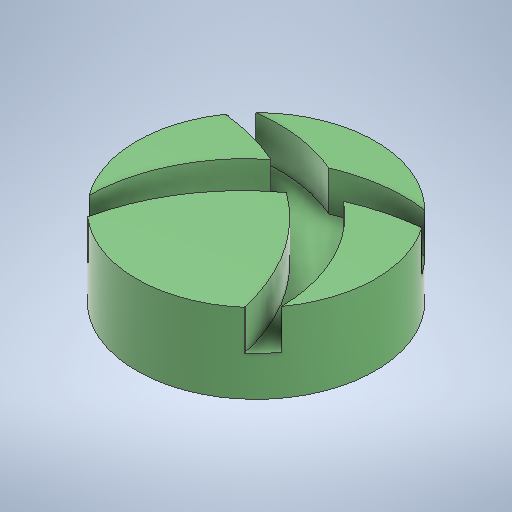
# Autodesk Inventor part: Xbox Simbol
Saved by Autodesk Inventor 2025 (Build 290162000, 162)
## iProperties
Created: 2024-06-12
Part Number: Xbox Simbol
Material: Genérico
Document SubType Name: Modeling
Designer: Eduardo Yuji
Density: 1 g/cm^3
Appearance: Padrão
Author: Eduardo Yuji
Autodesk Inventor part; units mm, degrees
ref_plane "YZ Plane" through (0, 0, 0) normal (1, 0, 0) x (0, 1, 0)
ref_plane "XZ Plane" through (0, 0, 0) normal (0, 1, 0) x (-1, 0, 0)
ref_plane "XY Plane" through (0, 0, 0) normal (0, 0, 1) x (1, 0, 0)
sketch "Esboço1" plane through (0, 0, 0) normal (0, 1, 0) x (-1, 0, 0)
  circle A0 centre (0, 0) radius 30
  constraints: 1 centre point, 1 coincident
extrude "Extrusão1" add sketch "Esboço1" along normal blind 20
sketch "Esboço2" plane through (0, 20, 0) normal (0, 1, 0) x (1, 0, 0)
  circle A0 centre (0, 0) radius 30 projected
  arc A1 (21.2132, 21.2132) -> (-24.1983, -17.7325) centre (15.7958, -18.4182) ccw
  arc A2 (24.1983, -17.7325) -> (-21.2132, 21.2132) centre (-15.7958, -18.4182) ccw
  arc A3 (24.688, 17.0441) -> (-19.7217, -22.6065) centre (20.2782, -22.7121) ccw
  arc A4 (19.7217, -22.6065) -> (-24.688, 17.0441) centre (-20.2782, -22.7121) ccw
  point P0 (-6.4534, 14.8229)
  point P1 (0, 11.7668)
  point P2 (6.4534, 14.8229)
  point P3 (0, 18.3308)
  constraints: 8 point on circle, 4 centre point, 9 other
extrude "Extrusão2" cut sketch "Esboço2" against normal blind 10 contours A3 A2 A1 A0 | A0 A4 A3 A2 | A3 A4 A1 A2 | A2 A1 A4 A0 | A3 A0 A1 A4
sketch "Esboço3" plane through (0, 20, 0) normal (0, 1, 0) x (1, 0, 0)
  circle A0 centre (0, 0) radius 30 projected
  arc A1 (-6.4534, 14.8229) -> (-24.688, 17.0441) centre (-20.2782, -22.7121) ccw projected
  arc A2 (19.733, -22.5966) -> (-24.688, 17.0441) centre (-29.6453, -33.2202) ccw
  arc A3 (24.688, 17.0441) -> (-19.733, -22.5966) centre (29.6453, -33.2202) ccw
  arc A4 (19.7217, -22.6065) -> (0, 11.7668) centre (-20.2782, -22.7121) ccw projected
  arc A5 (19.733, -22.5966) -> (0, 11.7668) centre (-9.6777, -16.638) ccw
  arc A6 (0, 11.7668) -> (-19.733, -22.5966) centre (6.925, -15.0573) ccw
  point P0 (0, 7.6727)
  point P1 (19.7215, -22.5432)
  constraints: 12 point on circle, 4 centre point
extrude "Extrusão3" cut sketch "Esboço3" against normal blind 10 contours A2 A3 A4 | A6 A2 A3 | A6 A4 A3 A2
sketch "Esboço4" plane through (0, 20, 0) normal (0, 1, 0) x (1, 0, 0)
  circle A0 centre (0, 0) radius 30 projected
  arc A1 (19.6815, -22.6415) -> (-24.7197, 16.9981) centre (-29.6674, -33.2312) ccw
  arc A2 (24.7197, 16.9981) -> (-19.6815, -22.6415) centre (29.6674, -33.2312) ccw
  arc A3 (24.7197, 16.9981) -> (-19.6815, -22.6415) centre (18.4995, -20.7217) ccw
  arc A4 (19.6815, -22.6415) -> (-24.7197, 16.9981) centre (-18.4995, -20.7217) ccw
  point P0 (3.9682, 10.2085)
  point P1 (0, 12.7334)
  point P2 (-3.9682, 10.2085)
  point P3 (0, 7.6014)
  constraints: 14 point on circle, 4 centre point
extrude "Extrusão4" cut sketch "Esboço4" against normal blind 10 contours A2 A4 A3 | A1 A2 A4 | A4 A3 A1 | A2 A1 A3 A4 | A3 A1 A2
